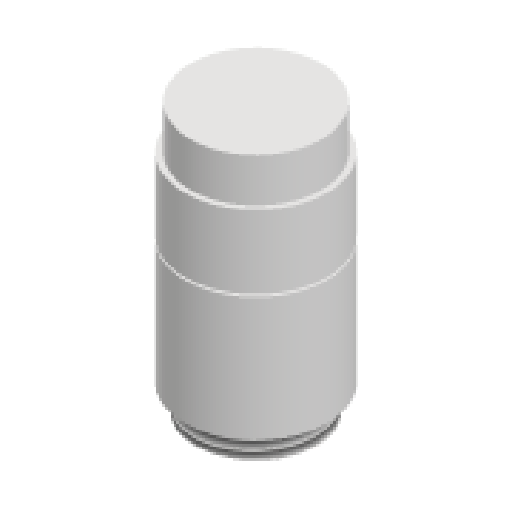
# Autodesk Inventor part: 00_CCTV_Lens_Hikvision_50mm_2.8
Saved by Autodesk Inventor 2024.1 (Build 281209000, 209)
## iProperties
Created: 2024-03-02
Part Number: 00_CCTV_Lens_Hikvision_50mm_2.8
Material: Generisch
Document SubType Name: Modeling
Designer: diederichbenedict
Density: 1 g/cm^3
Appearance: Vorgabe
Author: diederichbenedict
Autodesk Inventor part; units mm, degrees
ref_plane "YZ Plane" through (0, 0, 0) normal (1, 0, 0) x (0, 1, 0)
ref_plane "XZ Plane" through (0, 0, 0) normal (0, 1, 0) x (-1, 0, 0)
ref_plane "XY Plane" through (0, 0, 0) normal (0, 0, 1) x (1, 0, 0)
sketch "Skizze1" plane through (0, 0, 0) normal (0, 1, 0) x (-1, 0, 0)
  line L0 (0, 50) -> (13.5, 50)
  line L1 (13.5, 50) -> (13.5, 41)
  line L2 (13.5, 41) -> (14.6, 41)
  line L3 (14.6, 41) -> (14.6, 0)
  line L4 (14.6, 0) -> (0, 0)
  line L5 (0, 0) -> (0, 50)
  line L6 (14.6, 26) -> (13.6, 26)
  line L7 (13.6, 26) -> (13.6, 25.5)
  line L8 (13.6, 25.5) -> (14.6, 25.5)
  line L9 (14.6, 25.5) -> (14.6, 26)
  line L10 (0, 0) -> (13.95, 0)
  line L11 (13.95, 0) -> (13.95, -2.7)
  line L12 (13.95, -2.7) -> (0, -2.7)
  line L13 (0, -2.7) -> (0, 0)
  line L14 (0, -2.7) -> (12.5, -2.7)
  line L15 (12.5, -2.7) -> (12.5, -7.7)
  line L16 (12.5, -7.7) -> (0, -7.7)
  line L17 (0, -7.7) -> (0, -2.7)
  point P0 (14.1, 25.5)
  point P1 (13.6, 25.75)
  point P2 (14.1, 26)
  point P3 (14.05, 41)
  point P4 (13.95, 0)
  dimension "d0" = 13.5
  dimension "d1" = 9
  dimension "d2" = 90
  dimension "d3" = 1.1
  dimension "d4" = 270
  dimension "d5" = 0.5
  dimension "d6" = 1
  dimension "d7" = 15
  dimension "d9" = 13.95
  dimension "d10" = 2.7
  dimension "d13" = 12.5
  dimension "d14" = 5
  constraints: 36 end point, 8 perpendicular, 6 parallel, 4 horizontal, 4 midpoint, 1 point on line
  measures "d0" distance of L0.start L0.end
  measures "d1" distance of L0.end L1.end
  measures "d2" angle of L0 L1
  measures "d3" distance of L1.end L2.end
  measures "d5" distance from line of point (14.1, 25.5) L6
  measures "d6" distance from line of L3 point (13.6, 25.75)
  measures "d7" vertical distance of point (14.1, 26) point (14.05, 41)
  measures "d9" distance of L11.end L12.end
  measures "d10" distance of L10.end L11.end
  measures "d13" distance of L15.end L16.end
  measures "d14" distance of L14.end L15.end
revolve "Umdrehung1" add sketch "Skizze1" angle 360 about axis through (0, 0, 0) along (0, 0, 1) contours L0 L1 L2 L3 L6 L7 L8 L4 L5 | L4 L11 L12 L13 | L12 L15 L16 L17
thread "Gewinde1" size "M25x2" class "6g" standard "ANSI Metric M Profile" full length
